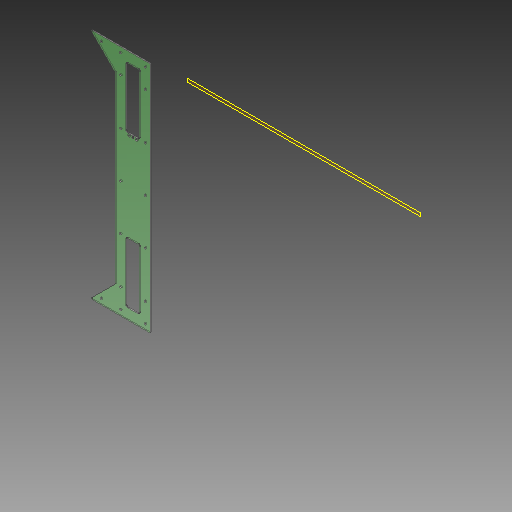
# Autodesk Inventor part: Acrylic-Back-Panel
Saved by Autodesk Inventor 2018 (Build 220112000, 112)
## iProperties
Created: 2016-07-14
Part Number: Acrylic-Back-Panel
Material: Polycarbonate, Clear
Document SubType Name: Modeling
Designer: User
Density: 1.2 g/cm^3
Appearance: Polycarbonate - Clear
Author: User
Autodesk Inventor part; units mm, degrees
(part 1 of 3)
ref_plane "YZ Plane" through (0, 0, 0) normal (1, 0, 0) x (0, 1, 0)
ref_plane "XZ Plane" through (0, 0, 0) normal (0, 1, 0) x (-1, 0, 0)
ref_plane "XY Plane" through (0, 0, 0) normal (0, 0, 1) x (1, 0, 0)
ref_plane "Work Plane1" through (-1999.0141, 29.8543, -2600.6334) normal (0, 0, 1) x (0, -1, 0)
sketch "Sketch1" plane through (-1999.0141, 29.8543, -2600.6334) normal (0, 0, 1) x (0, -1, 0)
  line L0 (7.3392, 781.9002) -> (682.3391, 781.9002)
  line L1 (682.3391, 781.9002) -> (682.3391, 281.9001)
  line L2 (682.3391, 281.9001) -> (7.3392, 281.9001)
  line L3 (7.3392, 281.9001) -> (7.3392, 781.9002)
  line L4 (7.3393, 781.9002) -> (-10.6607, 781.9002)
  line L5 (84.2338, 678.2351) -> (604.2338, 678.2351)
  line L6 (604.2338, 678.2351) -> (670.6983, 611.7707)
  line L7 (670.6983, 611.7707) -> (671.0121, 611.5131)
  line L8 (671.0121, 611.5131) -> (671.3702, 611.3217)
  line L9 (671.3702, 611.3217) -> (671.7587, 611.2039)
  line L10 (671.7587, 611.2039) -> (672.1627, 611.1641)
  line L11 (672.1627, 611.1641) -> (672.5668, 611.2039)
  line L12 (672.5668, 611.2039) -> (672.9553, 611.3217)
  line L13 (672.9553, 611.3217) -> (673.3134, 611.5131)
  line L14 (673.3134, 611.5131) -> (673.6272, 611.7707)
  line L15 (673.6272, 611.7707) -> (673.8848, 612.0845)
  line L16 (673.8848, 612.0845) -> (674.0761, 612.4426)
  line L17 (674.0761, 612.4426) -> (674.194, 612.8311)
  line L18 (674.194, 612.8311) -> (674.2338, 613.2351)
  line L19 (674.2338, 613.2351) -> (674.2338, 777.2351)
  line L20 (674.2338, 777.2351) -> (14.2338, 777.2351)
  line L21 (14.2338, 777.2351) -> (14.2338, 613.2351)
  line L22 (14.2338, 613.2351) -> (14.2736, 612.8311)
  line L23 (14.2736, 612.8311) -> (14.3915, 612.4426)
  line L24 (14.3915, 612.4426) -> (14.5828, 612.0845)
  line L25 (14.5828, 612.0845) -> (14.8404, 611.7707)
  line L26 (14.8404, 611.7707) -> (15.1542, 611.5131)
  line L27 (15.1542, 611.5131) -> (15.5123, 611.3217)
  line L28 (15.5123, 611.3217) -> (15.9008, 611.2039)
  line L29 (15.9008, 611.2039) -> (16.3049, 611.1641)
  line L30 (16.3049, 611.1641) -> (16.7089, 611.2039)
  line L31 (16.7089, 611.2039) -> (17.0974, 611.3217)
  line L32 (17.0974, 611.3217) -> (17.4555, 611.5131)
  line L33 (17.4555, 611.5131) -> (17.7693, 611.7707)
  line L34 (17.7693, 611.7707) -> (84.2338, 678.2351)
  line L35 (659.886, 760.801) -> (659.2338, 760.7151)
  line L36 (659.2338, 760.7151) -> (658.5816, 760.801)
  line L37 (658.5816, 760.801) -> (657.9738, 761.0528)
  line L38 (657.9738, 761.0528) -> (657.4519, 761.4532)
  line L39 (657.4519, 761.4532) -> (657.0514, 761.9751)
  line L40 (657.0514, 761.9751) -> (656.7997, 762.5829)
  line L41 (656.7997, 762.5829) -> (656.7138, 763.2351)
  line L42 (656.7138, 763.2351) -> (656.7997, 763.8874)
  line L43 (656.7997, 763.8874) -> (657.0514, 764.4951)
  line L44 (657.0514, 764.4951) -> (657.4519, 765.017)
  line L45 (657.4519, 765.017) -> (657.9738, 765.4175)
  line L46 (657.9738, 765.4175) -> (658.5816, 765.6693)
  line L47 (658.5816, 765.6693) -> (659.2338, 765.7551)
  line L48 (659.2338, 765.7551) -> (659.886, 765.6693)
  line L49 (659.886, 765.6693) -> (660.4938, 765.4175)
  line L50 (660.4938, 765.4175) -> (661.0157, 765.017)
  line L51 (661.0157, 765.017) -> (661.4162, 764.4951)
  line L52 (661.4162, 764.4951) -> (661.6679, 763.8874)
  line L53 (661.6679, 763.8874) -> (661.7538, 763.2351)
  line L54 (661.7538, 763.2351) -> (661.6679, 762.5829)
  line L55 (661.6679, 762.5829) -> (661.4162, 761.9751)
  line L56 (661.4162, 761.9751) -> (661.0157, 761.4532)
  line L57 (661.0157, 761.4532) -> (660.4938, 761.0528)
  line L58 (660.4938, 761.0528) -> (659.886, 760.801)
  line L59 (603.5816, 765.6693) -> (604.2338, 765.7551)
  line L60 (604.2338, 765.7551) -> (604.886, 765.6693)
  line L61 (604.886, 765.6693) -> (605.4938, 765.4175)
  line L62 (605.4938, 765.4175) -> (606.0157, 765.017)
  line L63 (606.0157, 765.017) -> (606.4162, 764.4951)
  line L64 (606.4162, 764.4951) -> (606.6679, 763.8874)
  line L65 (606.6679, 763.8874) -> (606.7538, 763.2351)
  line L66 (606.7538, 763.2351) -> (606.6679, 762.5829)
  line L67 (606.6679, 762.5829) -> (606.4162, 761.9751)
  line L68 (606.4162, 761.9751) -> (606.0157, 761.4532)
  line L69 (606.0157, 761.4532) -> (605.4938, 761.0528)
  line L70 (605.4938, 761.0528) -> (604.886, 760.801)
  line L71 (604.886, 760.801) -> (604.2338, 760.7151)
  line L72 (604.2338, 760.7151) -> (603.5816, 760.801)
  line L73 (603.5816, 760.801) -> (602.9738, 761.0528)
  line L74 (602.9738, 761.0528) -> (602.4519, 761.4532)
  line L75 (602.4519, 761.4532) -> (602.0514, 761.9751)
  line L76 (602.0514, 761.9751) -> (601.7997, 762.5829)
  line L77 (601.7997, 762.5829) -> (601.7138, 763.2351)
  line L78 (601.7138, 763.2351) -> (601.7997, 763.8874)
  line L79 (601.7997, 763.8874) -> (602.0514, 764.4951)
  line L80 (602.0514, 764.4951) -> (602.4519, 765.017)
  line L81 (602.4519, 765.017) -> (602.9738, 765.4175)
  line L82 (602.9738, 765.4175) -> (603.5816, 765.6693)
  line L83 (343.5816, 765.6693) -> (344.2338, 765.7551)
  line L84 (344.2338, 765.7551) -> (344.886, 765.6693)
  line L85 (344.886, 765.6693) -> (345.4938, 765.4175)
  line L86 (345.4938, 765.4175) -> (346.0157, 765.017)
  line L87 (346.0157, 765.017) -> (346.4162, 764.4951)
  line L88 (346.4162, 764.4951) -> (346.6679, 763.8874)
  line L89 (346.6679, 763.8874) -> (346.7538, 763.2351)
  line L90 (346.7538, 763.2351) -> (346.6679, 762.5829)
  line L91 (346.6679, 762.5829) -> (346.4162, 761.9751)
  line L92 (346.4162, 761.9751) -> (346.0157, 761.4532)
  line L93 (346.0157, 761.4532) -> (345.4938, 761.0528)
  line L94 (345.4938, 761.0528) -> (344.886, 760.801)
  line L95 (344.886, 760.801) -> (344.2338, 760.7151)
  line L96 (344.2338, 760.7151) -> (343.5816, 760.801)
  line L97 (343.5816, 760.801) -> (342.9738, 761.0528)
  line L98 (342.9738, 761.0528) -> (342.4519, 761.4532)
  line L99 (342.4519, 761.4532) -> (342.0514, 761.9751)
  line L100 (342.0514, 761.9751) -> (341.7996, 762.5829)
  line L101 (341.7996, 762.5829) -> (341.7138, 763.2351)
  line L102 (341.7138, 763.2351) -> (341.7996, 763.8874)
  line L103 (341.7996, 763.8874) -> (342.0514, 764.4951)
  line L104 (342.0514, 764.4951) -> (342.4519, 765.017)
  line L105 (342.4519, 765.017) -> (342.9738, 765.4175)
  line L106 (342.9738, 765.4175) -> (343.5816, 765.6693)
  line L107 (83.5816, 690.801) -> (82.9738, 691.0528)
  line L108 (82.9738, 691.0528) -> (82.4519, 691.4532)
  line L109 (82.4519, 691.4532) -> (82.0514, 691.9751)
  line L110 (82.0514, 691.9751) -> (81.7997, 692.5829)
  line L111 (81.7997, 692.5829) -> (81.7138, 693.2351)
  line L112 (81.7138, 693.2351) -> (81.7997, 693.8874)
  line L113 (81.7997, 693.8874) -> (82.0514, 694.4951)
  line L114 (82.0514, 694.4951) -> (82.4519, 695.0171)
  line L115 (82.4519, 695.0171) -> (82.9738, 695.4175)
  line L116 (82.9738, 695.4175) -> (83.5816, 695.6693)
  line L117 (83.5816, 695.6693) -> (84.2338, 695.7551)
  line L118 (84.2338, 695.7551) -> (84.886, 695.6693)
  line L119 (84.886, 695.6693) -> (85.4938, 695.4175)
  line L120 (85.4938, 695.4175) -> (86.0157, 695.0171)
  line L121 (86.0157, 695.0171) -> (86.4162, 694.4951)
  line L122 (86.4162, 694.4951) -> (86.6679, 693.8874)
  line L123 (86.6679, 693.8874) -> (86.7538, 693.2351)
  line L124 (86.7538, 693.2351) -> (86.6679, 692.5829)
  line L125 (86.6679, 692.5829) -> (86.4162, 691.9751)
  line L126 (86.4162, 691.9751) -> (86.0157, 691.4532)
  line L127 (86.0157, 691.4532) -> (85.4938, 691.0528)
  line L128 (85.4938, 691.0528) -> (84.886, 690.801)
  line L129 (84.886, 690.801) -> (84.2338, 690.7151)
  line L130 (84.2338, 690.7151) -> (83.5816, 690.801)
  line L131 (29.886, 635.801) -> (29.2338, 635.7152)
  line L132 (29.2338, 635.7152) -> (28.5816, 635.801)
  line L133 (28.5816, 635.801) -> (27.9738, 636.0528)
  line L134 (27.9738, 636.0528) -> (27.4519, 636.4532)
  line L135 (27.4519, 636.4532) -> (27.0514, 636.9751)
  line L136 (27.0514, 636.9751) -> (26.7997, 637.5829)
  line L137 (26.7997, 637.5829) -> (26.7138, 638.2351)
  line L138 (26.7138, 638.2351) -> (26.7997, 638.8874)
  line L139 (26.7997, 638.8874) -> (27.0514, 639.4951)
  line L140 (27.0514, 639.4951) -> (27.4519, 640.017)
  line L141 (27.4519, 640.017) -> (27.9738, 640.4175)
  line L142 (27.9738, 640.4175) -> (28.5816, 640.6693)
  line L143 (28.5816, 640.6693) -> (29.2338, 640.7551)
  line L144 (29.2338, 640.7551) -> (29.886, 640.6693)
  line L145 (29.886, 640.6693) -> (30.4938, 640.4175)
  line L146 (30.4938, 640.4175) -> (31.0157, 640.017)
  line L147 (31.0157, 640.017) -> (31.4162, 639.4951)
  line L148 (31.4162, 639.4951) -> (31.6679, 638.8874)
  line L149 (31.6679, 638.8874) -> (31.7538, 638.2351)
  line L150 (31.7538, 638.2351) -> (31.6679, 637.5829)
  line L151 (31.6679, 637.5829) -> (31.4162, 636.9751)
  line L152 (31.4162, 636.9751) -> (31.0157, 636.4532)
  line L153 (31.0157, 636.4532) -> (30.4938, 636.0528)
  line L154 (30.4938, 636.0528) -> (29.886, 635.801)
  line L155 (84.886, 760.801) -> (84.2338, 760.7151)
  line L156 (84.2338, 760.7151) -> (83.5816, 760.801)
  line L157 (83.5816, 760.801) -> (82.9738, 761.0528)
  line L158 (82.9738, 761.0528) -> (82.4519, 761.4532)
  line L159 (82.4519, 761.4532) -> (82.0514, 761.9751)
  line L160 (82.0514, 761.9751) -> (81.7997, 762.5829)
  line L161 (81.7997, 762.5829) -> (81.7138, 763.2351)
  line L162 (81.7138, 763.2351) -> (81.7997, 763.8874)
  line L163 (81.7997, 763.8874) -> (82.0514, 764.4951)
  line L164 (82.0514, 764.4951) -> (82.4519, 765.017)
  line L165 (82.4519, 765.017) -> (82.9738, 765.4175)
  line L166 (82.9738, 765.4175) -> (83.5816, 765.6693)
  line L167 (83.5816, 765.6693) -> (84.2338, 765.7551)
  line L168 (84.2338, 765.7551) -> (84.886, 765.6693)
  line L169 (84.886, 765.6693) -> (85.4938, 765.4175)
  line L170 (85.4938, 765.4175) -> (86.0157, 765.017)
  line L171 (86.0157, 765.017) -> (86.4162, 764.4951)
  line L172 (86.4162, 764.4951) -> (86.6679, 763.8874)
  line L173 (86.6679, 763.8874) -> (86.7538, 763.2351)
  line L174 (86.7538, 763.2351) -> (86.6679, 762.5829)
  line L175 (86.6679, 762.5829) -> (86.4162, 761.9751)
  line L176 (86.4162, 761.9751) -> (86.0157, 761.4532)
  line L177 (86.0157, 761.4532) -> (85.4938, 761.0528)
  line L178 (85.4938, 761.0528) -> (84.886, 760.801)
  line L179 (215.2838, 760.7151) -> (214.6316, 760.801)
  line L180 (214.6316, 760.801) -> (214.0238, 761.0528)
  line L181 (214.0238, 761.0528) -> (213.5019, 761.4532)
  line L182 (213.5019, 761.4532) -> (213.1014, 761.9751)
  line L183 (213.1014, 761.9751) -> (212.8497, 762.5829)
  line L184 (212.8497, 762.5829) -> (212.7638, 763.2351)
  line L185 (212.7638, 763.2351) -> (212.8497, 763.8874)
  line L186 (212.8497, 763.8874) -> (213.1014, 764.4951)
  line L187 (213.1014, 764.4951) -> (213.5019, 765.017)
  line L188 (213.5019, 765.017) -> (214.0238, 765.4175)
  line L189 (214.0238, 765.4175) -> (214.6316, 765.6693)
  line L190 (214.6316, 765.6693) -> (215.2838, 765.7551)
  line L191 (215.2838, 765.7551) -> (215.936, 765.6693)
  line L192 (215.936, 765.6693) -> (216.5438, 765.4175)
  line L193 (216.5438, 765.4175) -> (217.0657, 765.017)
  line L194 (217.0657, 765.017) -> (217.4662, 764.4951)
  line L195 (217.4662, 764.4951) -> (217.7179, 763.8874)
  line L196 (217.7179, 763.8874) -> (217.8038, 763.2351)
  line L197 (217.8038, 763.2351) -> (217.7179, 762.5829)
  line L198 (217.7179, 762.5829) -> (217.4662, 761.9751)
  line L199 (217.4662, 761.9751) -> (217.0657, 761.4532)
  line L200 (217.0657, 761.4532) -> (216.5438, 761.0528)
  line L201 (216.5438, 761.0528) -> (215.936, 760.801)
  line L202 (215.936, 760.801) -> (215.2838, 760.7151)
  line L203 (473.836, 760.801) -> (473.1838, 760.7151)
  line L204 (473.1838, 760.7151) -> (472.5316, 760.801)
  line L205 (472.5316, 760.801) -> (471.9238, 761.0528)
  line L206 (471.9238, 761.0528) -> (471.4019, 761.4532)
  line L207 (471.4019, 761.4532) -> (471.0014, 761.9751)
  line L208 (471.0014, 761.9751) -> (470.7497, 762.5829)
  line L209 (470.7497, 762.5829) -> (470.6638, 763.2351)
  line L210 (470.6638, 763.2351) -> (470.7497, 763.8874)
  line L211 (470.7497, 763.8874) -> (471.0014, 764.4951)
  line L212 (471.0014, 764.4951) -> (471.4019, 765.017)
  line L213 (471.4019, 765.017) -> (471.9238, 765.4175)
  line L214 (471.9238, 765.4175) -> (472.5316, 765.6693)
  line L215 (472.5316, 765.6693) -> (473.1838, 765.7551)
  line L216 (473.1838, 765.7551) -> (473.836, 765.6693)
  line L217 (473.836, 765.6693) -> (474.4438, 765.4175)
  line L218 (474.4438, 765.4175) -> (474.9657, 765.017)
  line L219 (474.9657, 765.017) -> (475.3662, 764.4951)
  line L220 (475.3662, 764.4951) -> (475.6179, 763.8874)
  line L221 (475.6179, 763.8874) -> (475.7038, 763.2351)
  line L222 (475.7038, 763.2351) -> (475.6179, 762.5829)
  line L223 (475.6179, 762.5829) -> (475.3662, 761.9751)
  line L224 (475.3662, 761.9751) -> (474.9657, 761.4532)
  line L225 (474.9657, 761.4532) -> (474.4438, 761.0528)
  line L226 (474.4438, 761.0528) -> (473.836, 760.801)
  line L227 (29.886, 760.801) -> (29.2338, 760.7151)
  line L228 (29.2338, 760.7151) -> (28.5816, 760.801)
  line L229 (28.5816, 760.801) -> (27.9738, 761.0528)
  line L230 (27.9738, 761.0528) -> (27.4519, 761.4532)
  line L231 (27.4519, 761.4532) -> (27.0514, 761.9751)
  line L232 (27.0514, 761.9751) -> (26.7997, 762.5829)
  line L233 (26.7997, 762.5829) -> (26.7138, 763.2351)
  line L234 (26.7138, 763.2351) -> (26.7997, 763.8874)
  line L235 (26.7997, 763.8874) -> (27.0514, 764.4951)
  line L236 (27.0514, 764.4951) -> (27.4519, 765.017)
  line L237 (27.4519, 765.017) -> (27.9738, 765.4175)
  line L238 (27.9738, 765.4175) -> (28.5816, 765.6693)
  line L239 (28.5816, 765.6693) -> (29.2338, 765.7551)
  line L240 (29.2338, 765.7551) -> (29.886, 765.6693)
  line L241 (29.886, 765.6693) -> (30.4938, 765.4175)
  line L242 (30.4938, 765.4175) -> (31.0157, 765.017)
  line L243 (31.0157, 765.017) -> (31.4162, 764.4951)
  line L244 (31.4162, 764.4951) -> (31.6679, 763.8874)
  line L245 (31.6679, 763.8874) -> (31.7538, 763.2351)
  line L246 (31.7538, 763.2351) -> (31.6679, 762.5829)
  line L247 (31.6679, 762.5829) -> (31.4162, 761.9751)
  line L248 (31.4162, 761.9751) -> (31.0157, 761.4532)
  line L249 (31.0157, 761.4532) -> (30.4938, 761.0528)
  line L250 (30.4938, 761.0528) -> (29.886, 760.801)
  line L251 (477.5812, 747.1924) -> (478.2338, 747.2351)
  line L252 (478.2338, 747.2351) -> (639.2338, 747.2351)
  line L253 (639.2338, 747.2351) -> (639.8864, 747.1924)
  line L254 (639.8864, 747.1924) -> (640.5279, 747.0648)
  line L255 (640.5279, 747.0648) -> (641.1472, 746.8545)
  line L256 (641.1472, 746.8545) -> (641.7338, 746.5653)
  line L257 (641.7338, 746.5653) -> (642.2776, 746.2019)
  line L258 (642.2776, 746.2019) -> (642.7693, 745.7707)
  line L259 (642.7693, 745.7707) -> (643.2006, 745.2789)
  line L260 (643.2006, 745.2789) -> (643.5639, 744.7351)
  line L261 (643.5639, 744.7351) -> (643.8532, 744.1486)
  line L262 (643.8532, 744.1486) -> (644.0634, 743.5292)
  line L263 (644.0634, 743.5292) -> (644.191, 742.8878)
  line L264 (644.191, 742.8878) -> (644.2338, 742.2351)
  line L265 (644.2338, 742.2351) -> (644.2338, 713.2351)
  line L266 (644.2338, 713.2351) -> (644.191, 712.5825)
  line L267 (644.191, 712.5825) -> (644.0634, 711.941)
  line L268 (644.0634, 711.941) -> (643.8532, 711.3217)
  line L269 (643.8532, 711.3217) -> (643.5639, 710.7351)
  line L270 (643.5639, 710.7351) -> (643.2006, 710.1913)
  line L271 (643.2006, 710.1913) -> (642.7693, 709.6996)
  line L272 (642.7693, 709.6996) -> (642.2776, 709.2684)
  line L273 (642.2776, 709.2684) -> (641.7338, 708.905)
  line L274 (641.7338, 708.905) -> (641.1472, 708.6157)
  line L275 (641.1472, 708.6157) -> (640.5279, 708.4055)
  line L276 (640.5279, 708.4055) -> (639.8864, 708.2779)
  line L277 (639.8864, 708.2779) -> (639.2338, 708.2351)
  line L278 (639.2338, 708.2351) -> (478.2338, 708.2351)
  line L279 (478.2338, 708.2351) -> (477.5812, 708.2779)
  line L280 (477.5812, 708.2779) -> (476.9397, 708.4055)
  line L281 (476.9397, 708.4055) -> (476.3204, 708.6157)
  line L282 (476.3204, 708.6157) -> (475.7338, 708.905)
  line L283 (475.7338, 708.905) -> (475.19, 709.2684)
  line L284 (475.19, 709.2684) -> (474.6983, 709.6996)
  line L285 (474.6983, 709.6996) -> (474.267, 710.1913)
  line L286 (474.267, 710.1913) -> (473.9037, 710.7351)
  line L287 (473.9037, 710.7351) -> (473.6144, 711.3217)
  line L288 (473.6144, 711.3217) -> (473.4042, 711.941)
  line L289 (473.4042, 711.941) -> (473.2766, 712.5825)
  line L290 (473.2766, 712.5825) -> (473.2338, 713.2351)
  line L291 (473.2338, 713.2351) -> (473.2338, 742.2351)
  line L292 (473.2338, 742.2351) -> (473.2766, 742.8878)
  line L293 (473.2766, 742.8878) -> (473.4042, 743.5292)
  line L294 (473.4042, 743.5292) -> (473.6144, 744.1486)
  line L295 (473.6144, 744.1486) -> (473.9037, 744.7351)
  line L296 (473.9037, 744.7351) -> (474.267, 745.2789)
  line L297 (474.267, 745.2789) -> (474.6983, 745.7707)
  line L298 (474.6983, 745.7707) -> (475.19, 746.2019)
  line L299 (475.19, 746.2019) -> (475.7338, 746.5653)
  line L300 (475.7338, 746.5653) -> (476.3204, 746.8545)
  line L301 (476.3204, 746.8545) -> (476.9397, 747.0648)
  line L302 (476.9397, 747.0648) -> (477.5812, 747.1924)
  line L303 (661.6679, 692.5829) -> (661.4162, 691.9751)
  line L304 (661.4162, 691.9751) -> (661.0157, 691.4532)
  line L305 (661.0157, 691.4532) -> (660.4938, 691.0528)
  line L306 (660.4938, 691.0528) -> (659.886, 690.801)
  line L307 (659.886, 690.801) -> (659.2338, 690.7151)
  line L308 (659.2338, 690.7151) -> (658.5816, 690.801)
  line L309 (658.5816, 690.801) -> (657.9738, 691.0528)
  line L310 (657.9738, 691.0528) -> (657.4519, 691.4532)
  line L311 (657.4519, 691.4532) -> (657.0514, 691.9751)
  line L312 (657.0514, 691.9751) -> (656.7997, 692.5829)
  line L313 (656.7997, 692.5829) -> (656.7138, 693.2351)
  line L314 (656.7138, 693.2351) -> (656.7997, 693.8874)
  line L315 (656.7997, 693.8874) -> (657.0514, 694.4951)
  line L316 (657.0514, 694.4951) -> (657.4519, 695.0171)
  line L317 (657.4519, 695.0171) -> (657.9738, 695.4175)
  line L318 (657.9738, 695.4175) -> (658.5816, 695.6693)
  line L319 (658.5816, 695.6693) -> (659.2338, 695.7551)
  line L320 (659.2338, 695.7551) -> (659.886, 695.6693)
  line L321 (659.886, 695.6693) -> (660.4938, 695.4175)
  line L322 (660.4938, 695.4175) -> (661.0157, 695.0171)
  line L323 (661.0157, 695.0171) -> (661.4162, 694.4951)
  line L324 (661.4162, 694.4951) -> (661.6679, 693.8874)
  line L325 (661.6679, 693.8874) -> (661.7538, 693.2351)
  line L326 (661.7538, 693.2351) -> (661.6679, 692.5829)
  line L327 (215.936, 690.801) -> (215.2838, 690.7151)
  line L328 (215.2838, 690.7151) -> (214.6316, 690.801)
  line L329 (214.6316, 690.801) -> (214.0238, 691.0528)
  line L330 (214.0238, 691.0528) -> (213.5019, 691.4532)
  line L331 (213.5019, 691.4532) -> (213.1014, 691.9751)
  line L332 (213.1014, 691.9751) -> (212.8497, 692.5829)
  line L333 (212.8497, 692.5829) -> (212.7638, 693.2351)
  line L334 (212.7638, 693.2351) -> (212.8497, 693.8874)
  line L335 (212.8497, 693.8874) -> (213.1014, 694.4951)
  line L336 (213.1014, 694.4951) -> (213.5019, 695.0171)
  line L337 (213.5019, 695.0171) -> (214.0238, 695.4175)
  line L338 (214.0238, 695.4175) -> (214.6316, 695.6693)
  line L339 (214.6316, 695.6693) -> (215.2838, 695.7551)
  line L340 (215.2838, 695.7551) -> (215.936, 695.6693)
  line L341 (215.936, 695.6693) -> (216.5438, 695.4175)
  line L342 (216.5438, 695.4175) -> (217.0657, 695.0171)
  line L343 (217.0657, 695.0171) -> (217.4662, 694.4951)
  line L344 (217.4662, 694.4951) -> (217.7179, 693.8874)
  line L345 (217.7179, 693.8874) -> (217.8038, 693.2351)
  line L346 (217.8038, 693.2351) -> (217.7179, 692.5829)
  line L347 (217.7179, 692.5829) -> (217.4662, 691.9751)
  line L348 (217.4662, 691.9751) -> (217.0657, 691.4532)
  line L349 (217.0657, 691.4532) -> (216.5438, 691.0528)
  line L350 (216.5438, 691.0528) -> (215.936, 690.801)
  line L351 (29.886, 690.801) -> (29.2338, 690.7151)
  line L352 (29.2338, 690.7151) -> (28.5816, 690.801)
  line L353 (28.5816, 690.801) -> (27.9738, 691.0528)
  line L354 (27.9738, 691.0528) -> (27.4519, 691.4532)
  line L355 (27.4519, 691.4532) -> (27.0514, 691.9751)
  line L356 (27.0514, 691.9751) -> (26.7997, 692.5829)
  line L357 (26.7997, 692.5829) -> (26.7138, 693.2351)
  line L358 (26.7138, 693.2351) -> (26.7997, 693.8874)
  line L359 (26.7997, 693.8874) -> (27.0514, 694.4951)
  line L360 (27.0514, 694.4951) -> (27.4519, 695.0171)
  line L361 (27.4519, 695.0171) -> (27.9738, 695.4175)
  line L362 (27.9738, 695.4175) -> (28.5816, 695.6693)
  line L363 (28.5816, 695.6693) -> (29.2338, 695.7551)
  line L364 (29.2338, 695.7551) -> (29.886, 695.6693)
  line L365 (29.886, 695.6693) -> (30.4938, 695.4175)
  line L366 (30.4938, 695.4175) -> (31.0157, 695.0171)
  line L367 (31.0157, 695.0171) -> (31.4162, 694.4951)
  line L368 (31.4162, 694.4951) -> (31.6679, 693.8874)
  line L369 (31.6679, 693.8874) -> (31.7538, 693.2351)
  line L370 (31.7538, 693.2351) -> (31.6679, 692.5829)
  line L371 (31.6679, 692.5829) -> (31.4162, 691.9751)
  line L372 (31.4162, 691.9751) -> (31.0157, 691.4532)
  line L373 (31.0157, 691.4532) -> (30.4938, 691.0528)
  line L374 (30.4938, 691.0528) -> (29.886, 690.801)
  line L375 (604.886, 690.801) -> (604.2338, 690.7151)
  line L376 (604.2338, 690.7151) -> (603.5816, 690.801)
  line L377 (603.5816, 690.801) -> (602.9738, 691.0528)
  line L378 (602.9738, 691.0528) -> (602.4519, 691.4532)
  line L379 (602.4519, 691.4532) -> (602.0514, 691.9751)
  line L380 (602.0514, 691.9751) -> (601.7997, 692.5829)
  line L381 (601.7997, 692.5829) -> (601.7138, 693.2351)
  line L382 (601.7138, 693.2351) -> (601.7997, 693.8874)
  line L383 (601.7997, 693.8874) -> (602.0514, 694.4951)
  line L384 (602.0514, 694.4951) -> (602.4519, 695.0171)
  line L385 (602.4519, 695.0171) -> (602.9738, 695.4175)
  line L386 (602.9738, 695.4175) -> (603.5816, 695.6693)
  line L387 (603.5816, 695.6693) -> (604.2338, 695.7551)
  line L388 (604.2338, 695.7551) -> (604.886, 695.6693)
  line L389 (604.886, 695.6693) -> (605.4938, 695.4175)
  line L390 (605.4938, 695.4175) -> (606.0157, 695.0171)
  line L391 (606.0157, 695.0171) -> (606.4162, 694.4951)
  line L392 (606.4162, 694.4951) -> (606.6679, 693.8874)
  line L393 (606.6679, 693.8874) -> (606.7538, 693.2351)
  line L394 (606.7538, 693.2351) -> (606.6679, 692.5829)
  line L395 (606.6679, 692.5829) -> (606.4162, 691.9751)
  line L396 (606.4162, 691.9751) -> (606.0157, 691.4532)
  line L397 (606.0157, 691.4532) -> (605.4938, 691.0528)
  line L398 (605.4938, 691.0528) -> (604.886, 690.801)
  line L399 (659.2338, 640.7551) -> (659.886, 640.6693)
  line L400 (659.886, 640.6693) -> (660.4938, 640.4175)
  line L401 (660.4938, 640.4175) -> (661.0157, 640.017)
  line L402 (661.0157, 640.017) -> (661.4162, 639.4951)
  line L403 (661.4162, 639.4951) -> (661.6679, 638.8874)
  line L404 (661.6679, 638.8874) -> (661.7538, 638.2351)
  line L405 (661.7538, 638.2351) -> (661.6679, 637.5829)
  line L406 (661.6679, 637.5829) -> (661.4162, 636.9751)
  line L407 (661.4162, 636.9751) -> (661.0157, 636.4532)
  line L408 (661.0157, 636.4532) -> (660.4938, 636.0528)
  line L409 (660.4938, 636.0528) -> (659.886, 635.801)
  line L410 (659.886, 635.801) -> (659.2338, 635.7152)
  line L411 (659.2338, 635.7152) -> (658.5816, 635.801)
  line L412 (658.5816, 635.801) -> (657.9738, 636.0528)
  line L413 (657.9738, 636.0528) -> (657.4519, 636.4532)
  line L414 (657.4519, 636.4532) -> (657.0514, 636.9751)
  line L415 (657.0514, 636.9751) -> (656.7997, 637.5829)
  line L416 (656.7997, 637.5829) -> (656.7138, 638.2351)
  line L417 (656.7138, 638.2351) -> (656.7997, 638.8874)
  line L418 (656.7997, 638.8874) -> (657.0514, 639.4951)
  line L419 (657.0514, 639.4951) -> (657.4519, 640.017)
  line L420 (657.4519, 640.017) -> (657.9738, 640.4175)
  line L421 (657.9738, 640.4175) -> (658.5816, 640.6693)
  line L422 (658.5816, 640.6693) -> (659.2338, 640.7551)
  line L423 (473.1838, 690.7151) -> (472.5316, 690.801)
  line L424 (472.5316, 690.801) -> (471.9238, 691.0528)
  line L425 (471.9238, 691.0528) -> (471.4019, 691.4532)
  line L426 (471.4019, 691.4532) -> (471.0014, 691.9751)
  line L427 (471.0014, 691.9751) -> (470.7497, 692.5829)
  line L428 (470.7497, 692.5829) -> (470.6638, 693.2351)
  line L429 (470.6638, 693.2351) -> (470.7497, 693.8874)
  line L430 (470.7497, 693.8874) -> (471.0014, 694.4951)
  line L431 (471.0014, 694.4951) -> (471.4019, 695.0171)
  line L432 (471.4019, 695.0171) -> (471.9238, 695.4175)
  line L433 (471.9238, 695.4175) -> (472.5316, 695.6693)
  line L434 (472.5316, 695.6693) -> (473.1838, 695.7551)
  line L435 (473.1838, 695.7551) -> (473.836, 695.6693)
  line L436 (473.836, 695.6693) -> (474.4438, 695.4175)
  line L437 (474.4438, 695.4175) -> (474.9657, 695.0171)
  line L438 (474.9657, 695.0171) -> (475.3662, 694.4951)
  line L439 (475.3662, 694.4951) -> (475.6179, 693.8874)
  line L440 (475.6179, 693.8874) -> (475.7038, 693.2351)
  line L441 (475.7038, 693.2351) -> (475.6179, 692.5829)
  line L442 (475.6179, 692.5829) -> (475.3662, 691.9751)
  line L443 (475.3662, 691.9751) -> (474.9657, 691.4532)
  line L444 (474.9657, 691.4532) -> (474.4438, 691.0528)
  line L445 (474.4438, 691.0528) -> (473.836, 690.801)
  line L446 (473.836, 690.801) -> (473.1838, 690.7151)
  line L447 (344.886, 690.801) -> (344.2338, 690.7151)
  line L448 (344.2338, 690.7151) -> (343.5816, 690.801)
  line L449 (343.5816, 690.801) -> (342.9738, 691.0528)
  line L450 (342.9738, 691.0528) -> (342.4519, 691.4532)
  line L451 (342.4519, 691.4532) -> (342.0514, 691.9751)
  line L452 (342.0514, 691.9751) -> (341.7996, 692.5829)
  line L453 (341.7996, 692.5829) -> (341.7138, 693.2351)
  line L454 (341.7138, 693.2351) -> (341.7996, 693.8874)
  line L455 (341.7996, 693.8874) -> (342.0514, 694.4951)
  line L456 (342.0514, 694.4951) -> (342.4519, 695.0171)
  line L457 (342.4519, 695.0171) -> (342.9738, 695.4175)
  line L458 (342.9738, 695.4175) -> (343.5816, 695.6693)
  line L459 (343.5816, 695.6693) -> (344.2338, 695.7551)
  line L460 (344.2338, 695.7551) -> (344.886, 695.6693)
  line L461 (344.886, 695.6693) -> (345.4938, 695.4175)
  line L462 (345.4938, 695.4175) -> (346.0157, 695.0171)
  line L463 (346.0157, 695.0171) -> (346.4162, 694.4951)
  line L464 (346.4162, 694.4951) -> (346.6679, 693.8874)
  line L465 (346.6679, 693.8874) -> (346.7538, 693.2351)
  line L466 (346.7538, 693.2351) -> (346.6679, 692.5829)
  line L467 (346.6679, 692.5829) -> (346.4162, 691.9751)
  line L468 (346.4162, 691.9751) -> (346.0157, 691.4532)
  line L469 (346.0157, 691.4532) -> (345.4938, 691.0528)
  line L470 (345.4938, 691.0528) -> (344.886, 690.801)
  line L471 (219.6024, 726.1038) -> (219.3482, 726.4351)
  line L472 (219.3482, 726.4351) -> (219.1883, 726.821)
  line L473 (219.1883, 726.821) -> (219.1338, 727.2351)
  line L474 (219.1338, 727.2351) -> (219.1883, 727.6493)
  line L475 (219.1883, 727.6493) -> (219.3482, 728.0351)
  line L476 (219.3482, 728.0351) -> (219.6024, 728.3665)
  line L477 (219.6024, 728.3665) -> (219.9338, 728.6208)
  line L478 (219.9338, 728.6208) -> (220.3197, 728.7806)
  line L479 (220.3197, 728.7806) -> (220.7338, 728.8351)
  line L480 (220.7338, 728.8351) -> (221.1479, 728.7806)
  line L481 (221.1479, 728.7806) -> (221.5338, 728.6208)
  line L482 (221.5338, 728.6208) -> (221.8651, 728.3665)
  line L483 (221.8651, 728.3665) -> (222.1194, 728.0351)
  line L484 (222.1194, 728.0351) -> (222.2793, 727.6493)
  line L485 (222.2793, 727.6493) -> (222.3338, 727.2351)
  line L486 (222.3338, 727.2351) -> (222.2793, 726.821)
  line L487 (222.2793, 726.821) -> (222.1194, 726.4351)
  line L488 (222.1194, 726.4351) -> (221.8651, 726.1038)
  line L489 (221.8651, 726.1038) -> (221.5338, 725.8495)
  line L490 (221.5338, 725.8495) -> (221.1479, 725.6896)
  line L491 (221.1479, 725.6896) -> (220.7338, 725.6351)
  line L492 (220.7338, 725.6351) -> (220.3197, 725.6896)
  line L493 (220.3197, 725.6896) -> (219.9338, 725.8495)
  line L494 (219.9338, 725.8495) -> (219.6024, 726.1038)
  line L495 (219.2338, 740.9244) -> (222.8338, 740.9244)
  line L496 (222.8338, 740.9244) -> (222.8338, 734.7244)
  line L497 (222.8338, 734.7244) -> (219.2338, 734.7244)
  line L498 (219.2338, 734.7244) -> (219.2338, 740.9244)
  line L499 (222.8338, 713.5244) -> (219.2338, 713.5244)
  line L500 (219.2338, 713.5244) -> (219.2338, 719.7244)
  line L501 (219.2338, 719.7244) -> (222.8338, 719.7244)
  line L502 (222.8338, 719.7244) -> (222.8338, 713.5244)
  line L503 (49.2338, 747.2351) -> (210.2338, 747.2351)
  line L504 (210.2338, 747.2351) -> (210.8864, 747.1924)
  line L505 (210.8864, 747.1924) -> (211.5279, 747.0648)
  line L506 (211.5279, 747.0648) -> (212.1472, 746.8545)
  line L507 (212.1472, 746.8545) -> (212.7338, 746.5653)
  line L508 (212.7338, 746.5653) -> (213.2776, 746.2019)
  line L509 (213.2776, 746.2019) -> (213.7693, 745.7707)
  line L510 (213.7693, 745.7707) -> (214.2006, 745.2789)
  line L511 (214.2006, 745.2789) -> (214.5639, 744.7351)
  line L512 (214.5639, 744.7351) -> (214.8532, 744.1486)
  line L513 (214.8532, 744.1486) -> (215.0634, 743.5292)
  line L514 (215.0634, 743.5292) -> (215.191, 742.8878)
  line L515 (215.191, 742.8878) -> (215.2338, 742.2351)
  line L516 (215.2338, 742.2351) -> (215.2338, 713.2351)
  line L517 (215.2338, 713.2351) -> (215.191, 712.5825)
  line L518 (215.191, 712.5825) -> (215.0634, 711.941)
  line L519 (215.0634, 711.941) -> (214.8532, 711.3217)
  line L520 (214.8532, 711.3217) -> (214.5639, 710.7351)
  line L521 (214.5639, 710.7351) -> (214.2006, 710.1913)
  line L522 (214.2006, 710.1913) -> (213.7693, 709.6996)
  line L523 (213.7693, 709.6996) -> (213.2776, 709.2684)
  line L524 (213.2776, 709.2684) -> (212.7338, 708.905)
  line L525 (212.7338, 708.905) -> (212.1472, 708.6157)
  line L526 (212.1472, 708.6157) -> (211.5279, 708.4055)
  line L527 (211.5279, 708.4055) -> (210.8864, 708.2779)
  line L528 (210.8864, 708.2779) -> (210.2338, 708.2351)
  line L529 (210.2338, 708.2351) -> (49.2338, 708.2351)
  line L530 (49.2338, 708.2351) -> (48.5812, 708.2779)
  line L531 (48.5812, 708.2779) -> (47.9397, 708.4055)
  line L532 (47.9397, 708.4055) -> (47.3204, 708.6157)
  line L533 (47.3204, 708.6157) -> (46.7338, 708.905)
  line L534 (46.7338, 708.905) -> (46.19, 709.2684)
  line L535 (46.19, 709.2684) -> (45.6983, 709.6996)
  line L536 (45.6983, 709.6996) -> (45.267, 710.1913)
  line L537 (45.267, 710.1913) -> (44.9037, 710.7351)
  line L538 (44.9037, 710.7351) -> (44.6144, 711.3217)
  line L539 (44.6144, 711.3217) -> (44.4042, 711.941)
  line L540 (44.4042, 711.941) -> (44.2766, 712.5825)
  line L541 (44.2766, 712.5825) -> (44.2338, 713.2351)
  line L542 (44.2338, 713.2351) -> (44.2338, 742.2351)
  line L543 (44.2338, 742.2351) -> (44.2766, 742.8878)
  line L544 (44.2766, 742.8878) -> (44.4042, 743.5292)
  line L545 (44.4042, 743.5292) -> (44.6144, 744.1486)
  line L546 (44.6144, 744.1486) -> (44.9037, 744.7351)
  line L547 (44.9037, 744.7351) -> (45.267, 745.2789)
  line L548 (45.267, 745.2789) -> (45.6983, 745.7707)
  line L549 (45.6983, 745.7707) -> (46.19, 746.2019)
  line L550 (46.19, 746.2019) -> (46.7338, 746.5653)
  line L551 (46.7338, 746.5653) -> (47.3204, 746.8545)
  line L552 (47.3204, 746.8545) -> (47.9397, 747.0648)
  line L553 (47.9397, 747.0648) -> (48.5812, 747.1924)
  line L554 (48.5812, 747.1924) -> (49.2338, 747.2351)
  point P0 (29.8543, 1999.0141)
  constraints: 1110 end point
extrude "Extrusion1" add sketch "Sketch1" along normal blind 3 contours L34 L33 L32 L31 L30 L29 L28 L27 L26 L25 L24 L23 L22 L21 L20 L19 L18 L17 L16 L15 L14 L13 L12 L11 L10 L9 L8 L7 L6 L5 | L503 L504 L505 L506 L507 L508 L509 L510 L511 L512 L513 L514 L515 L516 L517 L518 L519 L520 L521 L522 L523 L524 L525 L526 L527 L528 L529 L530 L531 L532 L533 L534 L535 L536 L537 L538 L539 L540 L541 L542 L543 L544 L545 L546 L547 L548 L549 L550 L551 L552 L553 L554
sketch "Sketch2" plane through (-1999.0141, 29.8543, -2600.6334) normal (0, 0, -1) x (-1, 0, 0)
  line L0 (-777.2351, -674.2338) -> (-777.2351, -14.2338) projected
  line L1 (-777.2351, -674.2338) -> (-777.2351, -14.2338) projected
  line L2 (-777.2351, -344.2338) -> (-709.0299, -344.2338)
  line L3 (-747.1924, -639.8864) -> (-747.2351, -639.2338)
  line L4 (-747.2351, -639.2338) -> (-747.2351, -478.2338)
  line L5 (-747.2351, -478.2338) -> (-747.1924, -477.5812)
  line L6 (-747.1924, -477.5812) -> (-747.0648, -476.9397)
  line L7 (-747.0648, -476.9397) -> (-746.8545, -476.3204)
  line L8 (-746.8545, -476.3204) -> (-746.5653, -475.7338)
  line L9 (-746.5653, -475.7338) -> (-746.2019, -475.19)
  line L10 (-746.2019, -475.19) -> (-745.7707, -474.6983)
  line L11 (-745.7707, -474.6983) -> (-745.2789, -474.267)
  line L12 (-745.2789, -474.267) -> (-744.7351, -473.9037)
  line L13 (-744.7351, -473.9037) -> (-744.1486, -473.6144)
  line L14 (-744.1486, -473.6144) -> (-743.5292, -473.4042)
  line L15 (-743.5292, -473.4042) -> (-742.8878, -473.2766)
  line L16 (-742.8878, -473.2766) -> (-742.2351, -473.2338)
  line L17 (-742.2351, -473.2338) -> (-713.2351, -473.2338)
  line L18 (-713.2351, -473.2338) -> (-712.5825, -473.2766)
  line L19 (-712.5825, -473.2766) -> (-711.941, -473.4042)
  line L20 (-711.941, -473.4042) -> (-711.3217, -473.6144)
  line L21 (-711.3217, -473.6144) -> (-710.7351, -473.9037)
  line L22 (-710.7351, -473.9037) -> (-710.1913, -474.267)
  line L23 (-710.1913, -474.267) -> (-709.6996, -474.6983)
  line L24 (-709.6996, -474.6983) -> (-709.2684, -475.19)
  line L25 (-709.2684, -475.19) -> (-708.905, -475.7338)
  line L26 (-708.905, -475.7338) -> (-708.6157, -476.3204)
  line L27 (-708.6157, -476.3204) -> (-708.4055, -476.9397)
  line L28 (-708.4055, -476.9397) -> (-708.2779, -477.5812)
  line L29 (-708.2779, -477.5812) -> (-708.2351, -478.2338)
  line L30 (-708.2351, -478.2338) -> (-708.2351, -639.2338)
  line L31 (-708.2351, -639.2338) -> (-708.2779, -639.8864)
  line L32 (-708.2779, -639.8864) -> (-708.4055, -640.5279)
  line L33 (-708.4055, -640.5279) -> (-708.6157, -641.1472)
  line L34 (-708.6157, -641.1472) -> (-708.905, -641.7338)
  line L35 (-708.905, -641.7338) -> (-709.2684, -642.2776)
  line L36 (-709.2684, -642.2776) -> (-709.6996, -642.7693)
  line L37 (-709.6996, -642.7693) -> (-710.1913, -643.2006)
  line L38 (-710.1913, -643.2006) -> (-710.7351, -643.5639)
  line L39 (-710.7351, -643.5639) -> (-711.3217, -643.8532)
  line L40 (-711.3217, -643.8532) -> (-711.941, -644.0634)
  line L41 (-711.941, -644.0634) -> (-712.5825, -644.191)
  line L42 (-712.5825, -644.191) -> (-713.2351, -644.2338)
  line L43 (-713.2351, -644.2338) -> (-742.2351, -644.2338)
  line L44 (-742.2351, -644.2338) -> (-742.8878, -644.191)
  line L45 (-742.8878, -644.191) -> (-743.5292, -644.0634)
  line L46 (-743.5292, -644.0634) -> (-744.1486, -643.8532)
  line L47 (-744.1486, -643.8532) -> (-744.7351, -643.5639)
  line L48 (-744.7351, -643.5639) -> (-745.2789, -643.2006)
  line L49 (-745.2789, -643.2006) -> (-745.7707, -642.7693)
  line L50 (-745.7707, -642.7693) -> (-746.2019, -642.2776)
  line L51 (-746.2019, -642.2776) -> (-746.5653, -641.7338)
  line L52 (-746.5653, -641.7338) -> (-746.8545, -641.1472)
  line L53 (-746.8545, -641.1472) -> (-747.0648, -640.5279)
  line L54 (-747.0648, -640.5279) -> (-747.1924, -639.8864)
  line L55 (-719.7244, -222.8338) -> (-719.7244, -219.2338) projected
  line L56 (-719.7244, -219.2338) -> (-713.5244, -219.2338) projected
  line L57 (-713.5244, -219.2338) -> (-713.5244, -222.8338) projected
  line L58 (-713.5244, -222.8338) -> (-719.7244, -222.8338) projected
  line L59 (-734.7244, -219.2338) -> (-734.7244, -222.8338) projected
  line L60 (-734.7244, -222.8338) -> (-740.9244, -222.8338) projected
  line L61 (-740.9244, -222.8338) -> (-740.9244, -219.2338) projected
  line L62 (-740.9244, -219.2338) -> (-734.7244, -219.2338) projected
  line L63 (-691.0528, -342.9738) -> (-690.801, -343.5816) projected
  line L64 (-690.801, -343.5816) -> (-690.7151, -344.2338) projected
  line L65 (-690.7151, -344.2338) -> (-690.801, -344.886) projected
  line L66 (-690.801, -344.886) -> (-691.0528, -345.4938) projected
  line L67 (-691.0528, -345.4938) -> (-691.4532, -346.0157) projected
  line L68 (-691.4532, -346.0157) -> (-691.9751, -346.4162) projected
  line L69 (-691.9751, -346.4162) -> (-692.5829, -346.6679) projected
  line L70 (-692.5829, -346.6679) -> (-693.2351, -346.7538) projected
  line L71 (-693.2351, -346.7538) -> (-693.8874, -346.6679) projected
  line L72 (-693.8874, -346.6679) -> (-694.4951, -346.4162) projected
  line L73 (-694.4951, -346.4162) -> (-695.0171, -346.0157) projected
  line L74 (-695.0171, -346.0157) -> (-695.4175, -345.4938) projected
  line L75 (-695.4175, -345.4938) -> (-695.6693, -344.886) projected
  line L76 (-695.6693, -344.886) -> (-695.7551, -344.2338) projected
  line L77 (-695.7551, -344.2338) -> (-695.6693, -343.5816) projected
  line L78 (-695.6693, -343.5816) -> (-695.4175, -342.9738) projected
  line L79 (-695.4175, -342.9738) -> (-695.0171, -342.4519) projected
  line L80 (-695.0171, -342.4519) -> (-694.4951, -342.0514) projected
  line L81 (-694.4951, -342.0514) -> (-693.8874, -341.7996) projected
  line L82 (-693.8874, -341.7996) -> (-693.2351, -341.7138) projected
  line L83 (-693.2351, -341.7138) -> (-692.5829, -341.7996) projected
  line L84 (-692.5829, -341.7996) -> (-691.9751, -342.0514) projected
  line L85 (-691.9751, -342.0514) -> (-691.4532, -342.4519) projected
  line L86 (-691.4532, -342.4519) -> (-691.0528, -342.9738) projected
  line L87 (-691.4532, -471.4019) -> (-691.0528, -471.9238) projected
  line L88 (-691.0528, -471.9238) -> (-690.801, -472.5316) projected
  line L89 (-690.801, -472.5316) -> (-690.7151, -473.1838) projected
  line L90 (-690.7151, -473.1838) -> (-690.801, -473.836) projected
  line L91 (-690.801, -473.836) -> (-691.0528, -474.4438) projected
  line L92 (-691.0528, -474.4438) -> (-691.4532, -474.9657) projected
  line L93 (-691.4532, -474.9657) -> (-691.9751, -475.3662) projected
  line L94 (-691.9751, -475.3662) -> (-692.5829, -475.6179) projected
  line L95 (-692.5829, -475.6179) -> (-693.2351, -475.7038) projected
  line L96 (-693.2351, -475.7038) -> (-693.8874, -475.6179) projected
  line L97 (-693.8874, -475.6179) -> (-694.4951, -475.3662) projected
  line L98 (-694.4951, -475.3662) -> (-695.0171, -474.9657) projected
  line L99 (-695.0171, -474.9657) -> (-695.4175, -474.4438) projected
  line L100 (-695.4175, -474.4438) -> (-695.6693, -473.836) projected
  line L101 (-695.6693, -473.836) -> (-695.7551, -473.1838) projected
  line L102 (-695.7551, -473.1838) -> (-695.6693, -472.5316) projected
  line L103 (-695.6693, -472.5316) -> (-695.4175, -471.9238) projected
  line L104 (-695.4175, -471.9238) -> (-695.0171, -471.4019) projected
  line L105 (-695.0171, -471.4019) -> (-694.4951, -471.0014) projected
  line L106 (-694.4951, -471.0014) -> (-693.8874, -470.7497) projected
  line L107 (-693.8874, -470.7497) -> (-693.2351, -470.6638) projected
  line L108 (-693.2351, -470.6638) -> (-692.5829, -470.7497) projected
  line L109 (-692.5829, -470.7497) -> (-691.9751, -471.0014) projected
  line L110 (-691.9751, -471.0014) -> (-691.4532, -471.4019) projected
  line L111 (-691.0528, -602.9738) -> (-690.801, -603.5816) projected
  line L112 (-690.801, -603.5816) -> (-690.7151, -604.2338) projected
  line L113 (-690.7151, -604.2338) -> (-690.801, -604.886) projected
  line L114 (-690.801, -604.886) -> (-691.0528, -605.4938) projected
  line L115 (-691.0528, -605.4938) -> (-691.4532, -606.0157) projected
  line L116 (-691.4532, -606.0157) -> (-691.9751, -606.4162) projected
  line L117 (-691.9751, -606.4162) -> (-692.5829, -606.6679) projected
  line L118 (-692.5829, -606.6679) -> (-693.2351, -606.7538) projected
  line L119 (-693.2351, -606.7538) -> (-693.8874, -606.6679) projected
  line L120 (-693.8874, -606.6679) -> (-694.4951, -606.4162) projected
  line L121 (-694.4951, -606.4162) -> (-695.0171, -606.0157) projected
  line L122 (-695.0171, -606.0157) -> (-695.4175, -605.4938) projected
  line L123 (-695.4175, -605.4938) -> (-695.6693, -604.886) projected
  line L124 (-695.6693, -604.886) -> (-695.7551, -604.2338) projected
  line L125 (-695.7551, -604.2338) -> (-695.6693, -603.5816) projected
  line L126 (-695.6693, -603.5816) -> (-695.4175, -602.9738) projected
  line L127 (-695.4175, -602.9738) -> (-695.0171, -602.4519) projected
  line L128 (-695.0171, -602.4519) -> (-694.4951, -602.0514) projected
  line L129 (-694.4951, -602.0514) -> (-693.8874, -601.7997) projected
  line L130 (-693.8874, -601.7997) -> (-693.2351, -601.7138) projected
  line L131 (-693.2351, -601.7138) -> (-692.5829, -601.7997) projected
  line L132 (-692.5829, -601.7997) -> (-691.9751, -602.0514) projected
  line L133 (-691.9751, -602.0514) -> (-691.4532, -602.4519) projected
  line L134 (-691.4532, -602.4519) -> (-691.0528, -602.9738) projected
  line L135 (-691.0528, -214.0238) -> (-690.801, -214.6316) projected
  line L136 (-690.801, -214.6316) -> (-690.7151, -215.2838) projected
  line L137 (-690.7151, -215.2838) -> (-690.801, -215.936) projected
  line L138 (-690.801, -215.936) -> (-691.0528, -216.5438) projected
  line L139 (-691.0528, -216.5438) -> (-691.4532, -217.0657) projected
  line L140 (-691.4532, -217.0657) -> (-691.9751, -217.4662) projected
  line L141 (-691.9751, -217.4662) -> (-692.5829, -217.7179) projected
  line L142 (-692.5829, -217.7179) -> (-693.2351, -217.8038) projected
  line L143 (-693.2351, -217.8038) -> (-693.8874, -217.7179) projected
  line L144 (-693.8874, -217.7179) -> (-694.4951, -217.4662) projected
  line L145 (-694.4951, -217.4662) -> (-695.0171, -217.0657) projected
  line L146 (-695.0171, -217.0657) -> (-695.4175, -216.5438) projected
  line L147 (-695.4175, -216.5438) -> (-695.6693, -215.936) projected
  line L148 (-695.6693, -215.936) -> (-695.7551, -215.2838) projected
  line L149 (-695.7551, -215.2838) -> (-695.6693, -214.6316) projected
  line L150 (-695.6693, -214.6316) -> (-695.4175, -214.0238) projected
  line L151 (-695.4175, -214.0238) -> (-695.0171, -213.5019) projected
  line L152 (-695.0171, -213.5019) -> (-694.4951, -213.1014) projected
  line L153 (-694.4951, -213.1014) -> (-693.8874, -212.8497) projected
  line L154 (-693.8874, -212.8497) -> (-693.2351, -212.7638) projected
  line L155 (-693.2351, -212.7638) -> (-692.5829, -212.8497) projected
  line L156 (-692.5829, -212.8497) -> (-691.9751, -213.1014) projected
  line L157 (-691.9751, -213.1014) -> (-691.4532, -213.5019) projected
  line L158 (-691.4532, -213.5019) -> (-691.0528, -214.0238) projected
  line L159 (-691.9751, -82.0514) -> (-691.4532, -82.4519) projected
  line L160 (-691.4532, -82.4519) -> (-691.0528, -82.9738) projected
  line L161 (-691.0528, -82.9738) -> (-690.801, -83.5816) projected
  line L162 (-690.801, -83.5816) -> (-690.7151, -84.2338) projected
  line L163 (-690.7151, -84.2338) -> (-690.801, -84.886) projected
  line L164 (-690.801, -84.886) -> (-691.0528, -85.4938) projected
  line L165 (-691.0528, -85.4938) -> (-691.4532, -86.0157) projected
  line L166 (-691.4532, -86.0157) -> (-691.9751, -86.4162) projected
  line L167 (-691.9751, -86.4162) -> (-692.5829, -86.6679) projected
  line L168 (-692.5829, -86.6679) -> (-693.2351, -86.7538) projected
  line L169 (-693.2351, -86.7538) -> (-693.8874, -86.6679) projected
  line L170 (-693.8874, -86.6679) -> (-694.4951, -86.4162) projected
  line L171 (-694.4951, -86.4162) -> (-695.0171, -86.0157) projected
  line L172 (-695.0171, -86.0157) -> (-695.4175, -85.4938) projected
  line L173 (-695.4175, -85.4938) -> (-695.6693, -84.886) projected
  line L174 (-695.6693, -84.886) -> (-695.7551, -84.2338) projected
  line L175 (-695.7551, -84.2338) -> (-695.6693, -83.5816) projected
  line L176 (-695.6693, -83.5816) -> (-695.4175, -82.9738) projected
  line L177 (-695.4175, -82.9738) -> (-695.0171, -82.4519) projected
  line L178 (-695.0171, -82.4519) -> (-694.4951, -82.0514) projected
  line L179 (-694.4951, -82.0514) -> (-693.8874, -81.7997) projected
  line L180 (-693.8874, -81.7997) -> (-693.2351, -81.7138) projected
  line L181 (-693.2351, -81.7138) -> (-692.5829, -81.7997) projected
  line L182 (-692.5829, -81.7997) -> (-691.9751, -82.0514) projected
  line L183 (-765.4175, -345.4938) -> (-765.6693, -344.886) projected
  line L184 (-765.6693, -344.886) -> (-765.7551, -344.2338) projected
  line L185 (-765.7551, -344.2338) -> (-765.6693, -343.5816) projected
  line L186 (-765.6693, -343.5816) -> (-765.4175, -342.9738) projected
  line L187 (-765.4175, -342.9738) -> (-765.017, -342.4519) projected
  line L188 (-765.017, -342.4519) -> (-764.4951, -342.0514) projected
  line L189 (-764.4951, -342.0514) -> (-763.8874, -341.7996) projected
  line L190 (-763.8874, -341.7996) -> (-763.2351, -341.7138) projected
  line L191 (-763.2351, -341.7138) -> (-762.5829, -341.7996) projected
  line L192 (-762.5829, -341.7996) -> (-761.9751, -342.0514) projected
  line L193 (-761.9751, -342.0514) -> (-761.4532, -342.4519) projected
  line L194 (-761.4532, -342.4519) -> (-761.0528, -342.9738) projected
  line L195 (-761.0528, -342.9738) -> (-760.801, -343.5816) projected
  line L196 (-760.801, -343.5816) -> (-760.7151, -344.2338) projected
  line L197 (-760.7151, -344.2338) -> (-760.801, -344.886) projected
  line L198 (-760.801, -344.886) -> (-761.0528, -345.4938) projected
  line L199 (-761.0528, -345.4938) -> (-761.4532, -346.0157) projected
  line L200 (-761.4532, -346.0157) -> (-761.9751, -346.4162) projected
  line L201 (-761.9751, -346.4162) -> (-762.5829, -346.6679) projected
  line L202 (-762.5829, -346.6679) -> (-763.2351, -346.7538) projected
  line L203 (-763.2351, -346.7538) -> (-763.8874, -346.6679) projected
  line L204 (-763.8874, -346.6679) -> (-764.4951, -346.4162) projected
  line L205 (-764.4951, -346.4162) -> (-765.017, -346.0157) projected
  line L206 (-765.017, -346.0157) -> (-765.4175, -345.4938) projected
  line L207 (-761.0528, -471.9238) -> (-760.801, -472.5316) projected
  line L208 (-760.801, -472.5316) -> (-760.7151, -473.1838) projected
  line L209 (-760.7151, -473.1838) -> (-760.801, -473.836) projected
  line L210 (-760.801, -473.836) -> (-761.0528, -474.4438) projected
  line L211 (-761.0528, -474.4438) -> (-761.4532, -474.9657) projected
  line L212 (-761.4532, -474.9657) -> (-761.9751, -475.3662) projected
  line L213 (-761.9751, -475.3662) -> (-762.5829, -475.6179) projected
  line L214 (-762.5829, -475.6179) -> (-763.2351, -475.7038) projected
  line L215 (-763.2351, -475.7038) -> (-763.8874, -475.6179) projected
  line L216 (-763.8874, -475.6179) -> (-764.4951, -475.3662) projected
  line L217 (-764.4951, -475.3662) -> (-765.017, -474.9657) projected
  line L218 (-765.017, -474.9657) -> (-765.4175, -474.4438) projected
  line L219 (-765.4175, -474.4438) -> (-765.6693, -473.836) projected
  line L220 (-765.6693, -473.836) -> (-765.7551, -473.1838) projected
  line L221 (-765.7551, -473.1838) -> (-765.6693, -472.5316) projected
  line L222 (-765.6693, -472.5316) -> (-765.4175, -471.9238) projected
  line L223 (-765.4175, -471.9238) -> (-765.017, -471.4019) projected
  line L224 (-765.017, -471.4019) -> (-764.4951, -471.0014) projected
  line L225 (-764.4951, -471.0014) -> (-763.8874, -470.7497) projected
  line L226 (-763.8874, -470.7497) -> (-763.2351, -470.6638) projected
  line L227 (-763.2351, -470.6638) -> (-762.5829, -470.7497) projected
  line L228 (-762.5829, -470.7497) -> (-761.9751, -471.0014) projected
  line L229 (-761.9751, -471.0014) -> (-761.4532, -471.4019) projected
  line L230 (-761.4532, -471.4019) -> (-761.0528, -471.9238) projected
  line L231 (-765.4175, -605.4938) -> (-765.6693, -604.886) projected
  line L232 (-765.6693, -604.886) -> (-765.7551, -604.2338) projected
  line L233 (-765.7551, -604.2338) -> (-765.6693, -603.5816) projected
  line L234 (-765.6693, -603.5816) -> (-765.4175, -602.9738) projected
  line L235 (-765.4175, -602.9738) -> (-765.017, -602.4519) projected
  line L236 (-765.017, -602.4519) -> (-764.4951, -602.0514) projected
  line L237 (-764.4951, -602.0514) -> (-763.8874, -601.7997) projected
  line L238 (-763.8874, -601.7997) -> (-763.2351, -601.7138) projected
  line L239 (-763.2351, -601.7138) -> (-762.5829, -601.7997) projected
  line L240 (-762.5829, -601.7997) -> (-761.9751, -602.0514) projected
  line L241 (-761.9751, -602.0514) -> (-761.4532, -602.4519) projected
  line L242 (-761.4532, -602.4519) -> (-761.0528, -602.9738) projected
  line L243 (-761.0528, -602.9738) -> (-760.801, -603.5816) projected
  line L244 (-760.801, -603.5816) -> (-760.7151, -604.2338) projected
  line L245 (-760.7151, -604.2338) -> (-760.801, -604.886) projected
  line L246 (-760.801, -604.886) -> (-761.0528, -605.4938) projected
  line L247 (-761.0528, -605.4938) -> (-761.4532, -606.0157) projected
  line L248 (-761.4532, -606.0157) -> (-761.9751, -606.4162) projected
  line L249 (-761.9751, -606.4162) -> (-762.5829, -606.6679) projected
  line L250 (-762.5829, -606.6679) -> (-763.2351, -606.7538) projected
  line L251 (-763.2351, -606.7538) -> (-763.8874, -606.6679) projected
  line L252 (-763.8874, -606.6679) -> (-764.4951, -606.4162) projected
  line L253 (-764.4951, -606.4162) -> (-765.017, -606.0157) projected
  line L254 (-765.017, -606.0157) -> (-765.4175, -605.4938) projected
  line L255 (-761.4532, -213.5019) -> (-761.0528, -214.0238) projected
  line L256 (-761.0528, -214.0238) -> (-760.801, -214.6316) projected
  line L257 (-760.801, -214.6316) -> (-760.7151, -215.2838) projected
  line L258 (-760.7151, -215.2838) -> (-760.801, -215.936) projected
  line L259 (-760.801, -215.936) -> (-761.0528, -216.5438) projected
  line L260 (-761.0528, -216.5438) -> (-761.4532, -217.0657) projected
  line L261 (-761.4532, -217.0657) -> (-761.9751, -217.4662) projected
  line L262 (-761.9751, -217.4662) -> (-762.5829, -217.7179) projected
  line L263 (-762.5829, -217.7179) -> (-763.2351, -217.8038) projected
  line L264 (-763.2351, -217.8038) -> (-763.8874, -217.7179) projected
  line L265 (-763.8874, -217.7179) -> (-764.4951, -217.4662) projected
  line L266 (-764.4951, -217.4662) -> (-765.017, -217.0657) projected
  line L267 (-765.017, -217.0657) -> (-765.4175, -216.5438) projected
  line L268 (-765.4175, -216.5438) -> (-765.6693, -215.936) projected
  line L269 (-765.6693, -215.936) -> (-765.7551, -215.2838) projected
  line L270 (-765.7551, -215.2838) -> (-765.6693, -214.6316) projected
  line L271 (-765.6693, -214.6316) -> (-765.4175, -214.0238) projected
  line L272 (-765.4175, -214.0238) -> (-765.017, -213.5019) projected
  line L273 (-765.017, -213.5019) -> (-764.4951, -213.1014) projected
  line L274 (-764.4951, -213.1014) -> (-763.8874, -212.8497) projected
  line L275 (-763.8874, -212.8497) -> (-763.2351, -212.7638) projected
  line L276 (-763.2351, -212.7638) -> (-762.5829, -212.8497) projected
  line L277 (-762.5829, -212.8497) -> (-761.9751, -213.1014) projected
  line L278 (-761.9751, -213.1014) -> (-761.4532, -213.5019) projected
  line L279 (-761.0528, -82.9738) -> (-760.801, -83.5816) projected
  line L280 (-760.801, -83.5816) -> (-760.7151, -84.2338) projected
  line L281 (-760.7151, -84.2338) -> (-760.801, -84.886) projected
  line L282 (-760.801, -84.886) -> (-761.0528, -85.4938) projected
  line L283 (-761.0528, -85.4938) -> (-761.4532, -86.0157) projected
  line L284 (-761.4532, -86.0157) -> (-761.9751, -86.4162) projected
  line L285 (-761.9751, -86.4162) -> (-762.5829, -86.6679) projected
  line L286 (-762.5829, -86.6679) -> (-763.2351, -86.7538) projected
  line L287 (-763.2351, -86.7538) -> (-763.8874, -86.6679) projected
  line L288 (-763.8874, -86.6679) -> (-764.4951, -86.4162) projected
  line L289 (-764.4951, -86.4162) -> (-765.017, -86.0157) projected
  line L290 (-765.017, -86.0157) -> (-765.4175, -85.4938) projected
  line L291 (-765.4175, -85.4938) -> (-765.6693, -84.886) projected
  line L292 (-765.6693, -84.886) -> (-765.7551, -84.2338) projected